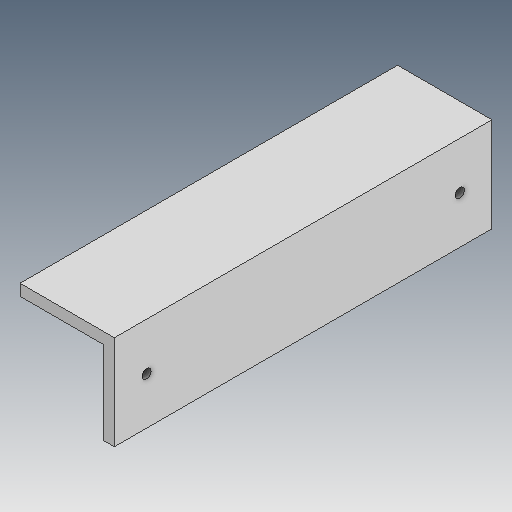
# Autodesk Inventor part: Halter vorne
Saved by Autodesk Inventor 2020 (Build 240168000, 168)
## iProperties
Created: 2021-06-29
Part Number: Halter vorne
Material: Generisch
Document SubType Name: Modeling
Designer: Mike
Density: 1 g/cm^3
Appearance: Vorgabe
Author: Mike
Autodesk Inventor part; units mm, degrees
ref_plane "YZ Plane" through (0, 0, 0) normal (1, 0, 0) x (0, 1, 0)
ref_plane "XZ Plane" through (0, 0, 0) normal (0, 1, 0) x (-1, 0, 0)
ref_plane "XY Plane" through (0, 0, 0) normal (0, 0, 1) x (1, 0, 0)
sketch "Skizze1" plane through (0, 0, 0) normal (0, 0, 1) x (1, 0, 0)
  line L0 (-10.271, 0) -> (24.729, 0) projected
  line L1 (0, -27.3364) -> (0, 7.6636) projected
  line L2 (16.729, -0.3364) -> (-5.271, -0.3364)
  line L3 (-5.271, -0.3364) -> (-5.271, 2.6636)
  line L4 (-5.271, 2.6636) -> (19.729, 2.6636)
  line L5 (19.729, 2.6636) -> (19.729, -22.3364)
  line L6 (19.729, -22.3364) -> (16.729, -22.3364)
  line L7 (16.729, -0.3364) -> (16.729, -22.3364)
  point P0 (0, 0)
  dimension "d0" = 3
  dimension "d1" = 3
  dimension "d2" = 25
  dimension "d3" = 25
  constraints: 12 end point, 4 perpendicular, 1 vertical
  measures "d0" distance between parallel lines of L5 L7
  measures "d1" distance between parallel lines of L4 L2
  measures "d2" distance of L4.end L5.end
  measures "d3" distance of L3.end L4.end
extrude "Extrusion1" add sketch "Skizze1" along normal blind 100
sketch "Skizze2" plane through (19.729, -22.3364, 0) normal (1, 0, 0) x (0, 0, -1)
  line L0 (0, 25) -> (-100, 25) projected
  line L1 (-100, 0) -> (-100, 25) projected
  line L2 (0, 0) -> (0, 25) projected
  point P0 (0, 22.3364)
  point P1 (-91.5, 12.5)
  point P2 (-8.5, 12.5)
  dimension "d6" = 12.5
  dimension "d7" = 12.5
  dimension "d8" = 8.5
  dimension "d9" = 8.5
  measures "d6" distance from line of L0 point (-8.5, 12.5)
  measures "d7" distance from line of L0 point (-91.5, 12.5)
  measures "d8" distance from line of L1 point (-91.5, 12.5)
  measures "d9" distance from line of L2 point (-8.5, 12.5)
hole "Bohrung1" at (19.729, -9.8364, 91.5) at (19.729, -9.8364, 8.5) direction (-1, 0, 0) diameter 2.459 depth 8.8 tip angle 118 thread size "M3x0.5" class "6H" standard "ISO Metric profile"
